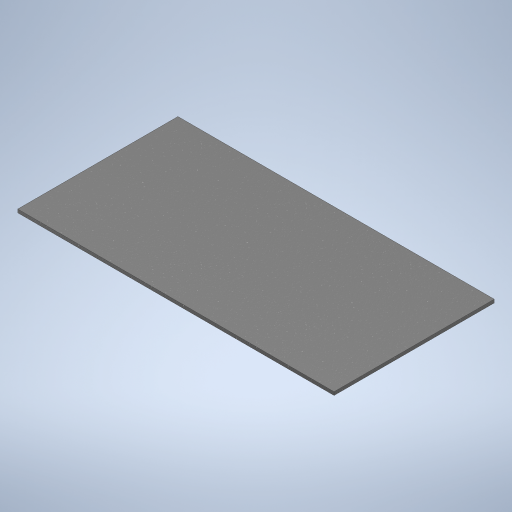
# Autodesk Inventor part: BottomOfTheBottomOfTheJukebox_Ocampo
Saved by Autodesk Inventor 2023 (Build 270158000, 158)
## iProperties
Created: 2025-03-05
Part Number: BottomOfTheBottomOfTheJukebox_Ocampo
Material: Generic
Document SubType Name: Modeling
Designer: FrameUser
Density: 1 g/cm^3
Appearance: Default
Author: FrameUser
Autodesk Inventor part; units mm, degrees
ref_plane "YZ Plane" through (0, 0, 0) normal (1, 0, 0) x (0, 1, 0)
ref_plane "XZ Plane" through (0, 0, 0) normal (0, 1, 0) x (-1, 0, 0)
ref_plane "XY Plane" through (0, 0, 0) normal (0, 0, 1) x (1, 0, 0)
sketch "Sketch4" plane through (0, 0, 0) normal (0, 1, 0) x (-1, 0, 0)
  line L0 (0, 0) -> (-614.3625, 0)
  line L1 (-614.3625, 0) -> (-614.3625, -311.15)
  line L2 (-614.3625, -311.15) -> (0, -311.15)
  line L3 (0, -311.15) -> (0, 0)
  dimension "d8" = 614.3625
  dimension "d9" = 311.15
  constraints: 8 end point, 3 perpendicular, 1 horizontal
  measures "d8" distance of L0.start L0.end
  measures "d9" distance of L0.end L1.end
extrude "Extrusion3" add sketch "Sketch4" along normal blind 6.35
body "Solid2"
